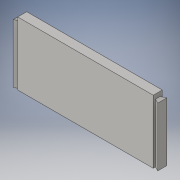
# Autodesk Inventor part: doveTailBar
Saved by Autodesk Inventor 2016 (Build 200138000, 138)
## iProperties
Created: 2015-11-04
Part Number: doveTailBar
Material: Generic
Document SubType Name: Modeling
Designer: rossmosier
Density: 1 g/cm^3
Appearance: Default
Author: rossmosier
Autodesk Inventor part; units mm, degrees
ref_plane "YZ Plane" through (0, 0, 0) normal (1, 0, 0) x (0, 1, 0)
ref_plane "XZ Plane" through (0, 0, 0) normal (0, 1, 0) x (-1, 0, 0)
ref_plane "XY Plane" through (0, 0, 0) normal (0, 0, 1) x (1, 0, 0)
sketch "Sketch1" plane through (0, 0, 0) normal (0, 1, 0) x (-1, 0, 0)
  line L0 (0, 0) -> (-190.5, 0)
  line L1 (-190.5, 0) -> (-190.5, -12.7)
  line L2 (-190.5, -12.7) -> (0, -12.7)
  line L3 (0, -12.7) -> (0, 0)
  dimension "d0" = 190.5
  dimension "d1" = 12.7
  constraints: 8 end point, 2 parallel, 1 horizontal, 1 perpendicular
  measures "d0" distance of L2.end L1.end
  measures "d1" distance of L1.end L0.end
extrude "Extrusion1" add sketch "Sketch1" along normal blind 88.9
sketch "Sketch2" plane through (0, 0, 0) normal (0, 1, 0) x (-1, 0, 0)
  line L0 (0, -12.7) -> (0, 0) construction
  line L1 (0, -12.6308) -> (0, 0) construction
  line L2 (0, -6.3154) -> (6.35, -6.3154) construction
  line L3 (6.35, 0) -> (6.35, -12.6308)
  line L4 (0, -6.3154) -> (0, -3.1658)
  line L5 (0, -6.3154) -> (0, -9.465)
  line L6 (0, -9.465) -> (6.35, -12.6308)
  line L7 (0, -3.1658) -> (6.35, 0)
  line L8 (-190.5, -12.7) -> (0, -12.7) construction
  line L9 (-95.25, -12.7) -> (-95.25, 0) construction
  line L10 (-190.5, -12.7) -> (-190.5, 0) construction
  line L11 (-196.85, 0) -> (-196.85, -12.6308)
  line L12 (-190.5, -9.465) -> (-196.85, -12.6308)
  line L13 (-190.5, -3.1658) -> (-196.85, 0)
  line L14 (-190.5, -9.465) -> (-190.5, -3.1658)
  line L15 (0, -9.465) -> (0, -3.1658)
  line L16 (-190.5, -9.465) -> (-196.85, -12.6308)
  line L17 (-196.85, 0) -> (-190.5, -3.1658)
  dimension "d4" = 6.35
  dimension "d5" = 3.1496
  dimension "d6" = 3.1496
  constraints: 32 end point, 5 symmetric about line, 3 collinear, 3 point on line, 3 vertical, 2 midpoint, 1 horizontal
  measures "d4" distance of L2.start L2.end
  measures "d5" distance of L2.start L4.end
  measures "d6" distance of L2.start L5.end
extrude "Extrusion2" add sketch "Sketch2" along normal blind 82.55
body "Solid1"
